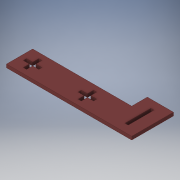
# Autodesk Inventor part: Brazo_Inferior
Saved by Autodesk Inventor 2019 (Build 230136000, 136)
## iProperties
Created: 2020-02-09
Part Number: Brazo_Inferior
Material: Generic
Document SubType Name: Modeling
Designer: Omar
Density: 1 g/cm^3
Appearance: Default
Author: Omar
Autodesk Inventor part; units mm, degrees
ref_plane "YZ Plane" through (0, 0, 0) normal (1, 0, 0) x (0, 1, 0)
ref_plane "XZ Plane" through (0, 0, 0) normal (0, 1, 0) x (-1, 0, 0)
ref_plane "XY Plane" through (0, 0, 0) normal (0, 0, 1) x (1, 0, 0)
sketch "Sketch1" plane through (0, 0, 0) normal (0, 1, 0) x (-1, 0, 0)
  line L0 (-1.59, 12.5) -> (1.59, 12.5)
  line L1 (1.59, 12.5) -> (1.59, -12.5)
  line L2 (1.59, -12.5) -> (-1.59, -12.5)
  line L3 (-1.59, -12.5) -> (-1.59, 12.5)
  line L4 (-1.59, 12.5) -> (1.59, -12.5) construction
  line L5 (1.59, 12.5) -> (-1.59, -12.5) construction
  line L6 (12.5, 20) -> (-12.5, 20)
  line L7 (-12.5, 20) -> (-12.5, -20)
  line L8 (-12.5, -20) -> (12.5, -20)
  line L9 (12.5, -20) -> (12.5, 20)
  line L10 (12.5, 20) -> (107.5, 20)
  line L11 (107.5, 20) -> (107.5, -5)
  line L12 (107.5, -5) -> (12.5, -5)
  line L13 (12.5, -5) -> (12.5, 20)
  line L14 (107.5, 20) -> (82.5, 20)
  line L15 (88.91, 20) -> (92.09, 20)
  line L16 (102.5, 9.09) -> (87.5, 9.09)
  line L17 (87.5, 9.09) -> (87.5, 5.91)
  line L18 (87.5, 5.91) -> (102.5, 5.91)
  line L19 (102.5, 5.91) -> (102.5, 9.09)
  line L20 (96.59, 15) -> (93.41, 15)
  line L21 (93.41, 15) -> (93.41, 0)
  line L22 (93.41, 0) -> (96.59, 0)
  line L23 (96.59, 0) -> (96.59, 15)
  line L24 (96.59, 15) -> (93.41, 0) construction
  line L25 (93.41, 15) -> (96.59, 0) construction
  line L26 (50, 9.09) -> (35, 9.09)
  line L27 (35, 9.09) -> (35, 5.91)
  line L28 (35, 5.91) -> (50, 5.91)
  line L29 (50, 5.91) -> (50, 9.09)
  line L30 (44.09, 15) -> (40.91, 15)
  line L31 (40.91, 15) -> (40.91, 0)
  line L32 (40.91, 0) -> (44.09, 0)
  line L33 (44.09, 0) -> (44.09, 15)
  line L34 (44.09, 15) -> (40.91, 0) construction
  line L35 (40.91, 15) -> (44.09, 0) construction
  point P0 (0, 0)
  point P1 (95, 7.5)
  point P2 (42.5, 7.5)
  dimension "d0" = 3.18
  dimension "d1" = 25
  dimension "d2" = 25
  dimension "d3" = 12.5
  dimension "d4" = 20
  dimension "d5" = 20
  dimension "d6" = 95
  dimension "d7" = 25
  dimension "d35" = 15
  dimension "d36" = 3.18
  dimension "d38" = 3.18
  dimension "d39" = 15
  dimension "d40" = 7.5
  dimension "d41" = 1.59
  dimension "d42" = 12.5
  dimension "d43" = 12.5
  dimension "d44" = 15
  dimension "d45" = 3.18
  dimension "d46" = 3.18
  dimension "d47" = 15
  dimension "d48" = 7.5
  dimension "d49" = 1.59
  dimension "d50" = 30
  dimension "d51" = 12.5
  constraints: 72 end point, 14 parallel, 8 horizontal, 7 perpendicular, 6 midpoint
  measures "d0" distance of L1.end L2.end
  measures "d1" distance of L0.end L1.end
  measures "d2" distance of L7.end L8.end
  measures "d3" distance from line of point (0, 0) L9
  measures "d4" distance from line of L8 point (0, 0)
  measures "d5" distance from line of L6 point (0, 0)
  measures "d6" distance of L11.end L12.end
  measures "d7" distance of L10.end L11.end
  measures "d35" distance of L18.end L17.end
  measures "d36" distance of L17.end L16.end
  measures "d38" distance of L22.end L21.end
  measures "d39" distance of L21.end L20.end
  measures "d40" distance from line of L19 point (95, 7.5)
  measures "d41" distance from line of L18 point (95, 7.5)
  measures "d42" distance from line of L12 point (95, 7.5)
  measures "d43" distance from line of L11 point (95, 7.5)
  measures "d44" distance of L28.end L27.end
  measures "d45" distance of L27.end L27.start
  measures "d46" distance of L32.end L31.end
  measures "d47" distance of L31.end L30.end
  measures "d48" distance from line of L29 point (42.5, 7.5)
  measures "d49" distance from line of L28 point (42.5, 7.5)
  measures "d50" distance from line of L9 point (42.5, 7.5)
  measures "d51" distance from line of L10 point (42.5, 7.5)
extrude "Extrusion2" add sketch "Sketch1" along normal blind 3.18
body "Solid2"
